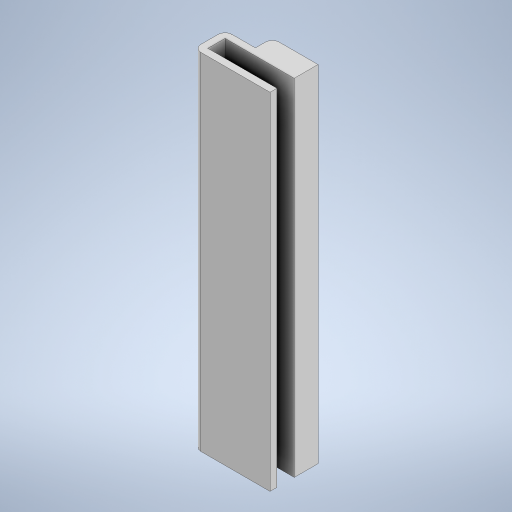
# Autodesk Inventor part: magnet
Saved by Autodesk Inventor 2024 (Build 280153000, 153)
## iProperties
Created: 2024-01-25
Part Number: magnet
Material: Generic
Document SubType Name: Modeling
Designer: Luke.Macenski3281
Density: 1 g/cm^3
Appearance: Default
Author: Luke.Macenski3281
Autodesk Inventor part; units mm, degrees
ref_plane "YZ Plane" through (0, 0, 0) normal (1, 0, 0) x (0, 1, 0)
ref_plane "XZ Plane" through (0, 0, 0) normal (0, 1, 0) x (-1, 0, 0)
ref_plane "XY Plane" through (0, 0, 0) normal (0, 0, 1) x (1, 0, 0)
sketch "Sketch1" plane through (0, 0, 0) normal (0, 1, 0) x (-1, 0, 0)
  line L0 (0, 0) -> (25.4, 0)
  line L1 (25.4, 0) -> (25.4, 2.54)
  line L2 (25.4, 2.54) -> (0, 2.54)
  line L3 (0, 2.54) -> (0, 0)
  line L4 (25.4, 2.54) -> (27.94, 2.54)
  line L5 (27.94, 2.54) -> (27.94, -8.89)
  line L6 (27.94, -8.89) -> (25.4, -8.89)
  line L7 (25.4, -8.89) -> (25.4, 2.54)
  line L8 (-1.2994, 2.54) -> (27.94, 2.54)
  line L9 (25.4, -8.89) -> (0, -8.89)
  line L10 (0, -8.89) -> (0, -6.35)
  line L11 (0, -6.35) -> (25.4, -6.35)
  line L12 (25.4, -6.35) -> (25.4, -8.89)
  line L13 (8.3183, -8.89) -> (0, -8.89)
  line L14 (0, -8.89) -> (0, -12.3973)
  line L15 (0, -12.3973) -> (8.3183, -12.3973)
  line L16 (8.3183, -12.3973) -> (8.3183, -8.89)
  line L17 (0, -12.3973) -> (0, -6.35)
  line L18 (8.3183, -12.3973) -> (16.7954, -12.3973)
  line L19 (16.7954, -12.3973) -> (16.7954, -8.89)
  line L20 (16.7954, -8.89) -> (8.3183, -8.89)
  line L21 (8.3183, -8.89) -> (8.3183, -12.3973)
  line L22 (0, -12.3973) -> (16.7954, -12.3973)
  line L23 (16.7954, -12.3973) -> (16.7954, -15.1027)
  line L24 (16.7954, -15.1027) -> (0, -15.1027)
  line L25 (0, -15.1027) -> (0, -12.3973)
  point P0 (26.67, 2.54)
  point P1 (26.67, -8.89)
  point P2 (0, -8.89)
  point P3 (0, -8.89)
  dimension "d0" = 25.4
  dimension "d1" = 2.54
  dimension "d2" = 2.54
  dimension "d3" = 11.43
  dimension "d4" = 2.54
  constraints: 52 end point, 12 parallel, 6 horizontal, 6 perpendicular, 4 point on line, 2 midpoint
  measures "d0" distance of L2.end L1.end
  measures "d1" distance between parallel lines of L0 L2
  measures "d2" distance of L5.end L6.end
  measures "d3" distance of point (26.67, 2.54) point (26.67, -8.89)
  measures "d4" distance between parallel lines of L9 L11
extrude "Extrusion1" add sketch "Sketch1" along normal blind 127
sketch "Sketch4" plane through (0, 0, -15.1027) normal (0, 0, -1) x (-1, 0, 0)
  circle A0 centre (8.4134, 114.3) radius 4.95
  line L0 (16.7954, 0) -> (16.7954, 127) projected
  circle A1 centre (8.4134, 88.9) radius 4.95
  circle A2 centre (8.4134, 63.5) radius 4.95
  circle A3 centre (8.4134, 38.1) radius 4.95
  circle A4 centre (8.4134, 12.7) radius 4.95
  line L1 (0, 127) -> (16.7954, 127) projected
  point P0 (0, 0)
  dimension "d15" = 9.9
  dimension "d16" = 8.382
  dimension "d19" = 25.4
  dimension "d24" = 12.7
  constraints: 5 centre point, 1 vertical, 8 other
  measures "d15" diameter of A0
  measures "d16" distance from line of L0 A0.centre
  measures "d19" distance of A0.centre A1.centre
  measures "d24" distance from line of L1 A0.centre
extrude "Extrusion3" cut sketch "Sketch4" against normal blind 3
fillet "Fillet3" radius 2.54 3 edges at (-27.94, 63.5, -8.89) (-27.94, 63.5, 2.54) (-16.7954, 63.5, -15.1027)
body "Solid1"
